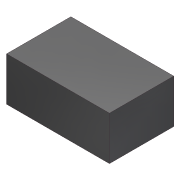
# Autodesk Inventor part: thermistor_0805
Saved by Autodesk Inventor 2014 SP1 (Build 180222100, 222)
## iProperties
Created: 2012-11-09
Document SubType Name: Modeling
Designer: Robert Davis
Density: 2.11 g/cm^3
Description: THERMISTOR, 0805
Material: SMT (95% LCP, 5% PhosBr)
Mass: 0.00448375 g
Surface Area: 0.10525 cm^2
Volume: 0.002125 cm^3
Appearance: Smooth - Medium Gray
Author: Robert Davis
Autodesk Inventor part; units mm, degrees
ref_plane "YZ Plane" through (0, 0, 0) normal (1, 0, 0) x (0, 1, 0)
ref_plane "XZ Plane" through (0, 0, 0) normal (0, 1, 0) x (-1, 0, 0)
ref_plane "XY Plane" through (0, 0, 0) normal (0, 0, 1) x (1, 0, 0)
sketch "Sketch1" plane through (0, 0, 0) normal (0, 0, 1) x (1, 0, 0)
  line L0 (-1, 0.625) -> (1, 0.625)
  line L1 (1, 0.625) -> (1, -0.625)
  line L2 (1, -0.625) -> (-1, -0.625)
  line L3 (-1, -0.625) -> (-1, 0.625)
  line L4 (0, 0) -> (0.5967, 0)
  line L5 (0, 0) -> (0, 0.6476)
  dimension "d0" = 2
  dimension "d1" = 1.25
  constraints: 12 end point, 3 horizontal, 3 vertical, 1 coincident, 2 other
  measures "d0" distance of L0.start L0.end
  measures "d1" distance of L0.end L1.end
extrude "Extrusion1" add sketch "Sketch1" along normal blind 0.85
body "Solid1"
